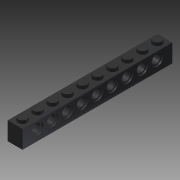
# Autodesk Inventor part: LEGO Technic Brick 1x10 with Holes
Saved by Autodesk Inventor 2013 (Build 170138000, 138)
## iProperties
Created: 2013-06-01
Part Number: LEGO Technic Brick 1x10 with Holes
Material: Generic
Document SubType Name: Modeling
Designer: Masta
Density: 1 g/cm^3
Author: Masta
Autodesk Inventor part; units mm, degrees
ref_plane "YZ Plane" through (0, 0, 0) normal (1, 0, 0) x (0, 1, 0)
ref_plane "XZ Plane" through (0, 0, 0) normal (0, 1, 0) x (-1, 0, 0)
sketch "Sketch1" plane through (0, 0, 0) normal (0, 0, 1) x (1, 0, 0)
  line L0 (-4, -4) -> (4, -4)
  line L1 (4, -4) -> (4, 4)
  line L2 (4, 4) -> (-4, 4)
  line L3 (-4, 4) -> (-4, -4)
  line L4 (-4, -4) -> (4, 4) construction
  line L5 (4, -4) -> (-4, 4) construction
  circle A0 centre (0, 0) radius 2.4
  dimension "d0" = 8
  dimension "d1" = 8
  dimension "d2" = 4.8
  constraints: 12 end point, 2 midpoint, 2 parallel, 1 centre point, 1 coincident, 1 horizontal, 1 perpendicular
  measures "d0" distance of L2.end L1.end
  measures "d1" distance of L1.end L0.end
  measures "d2" diameter of A0
extrude "Extrusion1" add sketch "Sketch1" along normal blind 9.6 contours L3 L2 L1 L0 | A0
extrude "Extrusion2" add sketch "Sketch1" along normal blind 11.3 contours A0
extrude "Extrusion3" cut sketch "Sketch1" along normal blind 1.7 contours A0
pattern_linear "Rectangular Pattern1" count 10 spacing 8 along (0, 1, 0) of "Extrusion1", "Extrusion2", "Extrusion3"
sketch "Sketch2" plane through (4, -4, 9.6) normal (1, 0, 0) x (0, 0, -1)
  circle A0 centre (4, 8) radius 2.4
  circle A1 centre (4, 8) radius 3.1
  line L0 (9.6, 0) -> (9.6, 80) projected
  line L1 (9.6, 0) -> (0, 0) projected
  point P0 (9.6, 4)
  dimension "d12" = 4.8
  dimension "d14" = 6.2
  dimension "d22" = 8
  dimension "d23" = 5.6
  constraints: 2 centre point, 1 coincident
  measures "d12" diameter of A0
  measures "d14" diameter of A1
  measures "d22" distance from line of L1 A0.centre
  measures "d23" distance from line of A0.centre L0
ref_plane "Work Plane1" through (0, -4, 9.6) normal (1, 0, 0) x (0, 0, -1)
extrude "Extrusion4" cut sketch "Sketch2" against normal up to next contours A0
extrude "Extrusion5" cut sketch "Sketch2" against normal blind 0.8
mirror "Mirror1" about plane through (0, -4, 9.6) normal (1, 0, 0) of "Extrusion5"
pattern_linear "Rectangular Pattern2" count 9 spacing 8 along (0, 1, 0) of "Extrusion4", "Extrusion5", "Mirror1"
equation "\"d11\" = d0"
equation "\"d21\" = d0"
body "Solid1"
